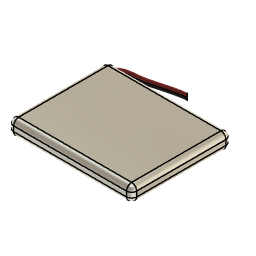
Bobblestat_rev2_v22 (Autodesk Fusion 360 archive; units mm, degrees)
design "LiPo Battery Dummy"
Autodesk Fusion 360 part; units mm, degrees
sketch "Sketch1" plane through (0, 0, 0) normal (0, 0, 1) x (1, 0, 0)
  line L0 (0, 0) -> (36.5, 0)
  line L1 (36.5, 0) -> (36.5, 29.5)
  line L2 (36.5, 29.5) -> (0, 29.5)
  line L3 (0, 29.5) -> (0, 0)
  dimension "d1" = 36.5
  dimension "d2" = 29.5
  constraint horizontal L0
  constraint vertical L1
  constraint horizontal L2
  constraint vertical L3
  constraint coincident L0.start L3.end
  measures "d1" distance of L0.start L0.end
  measures "d2" distance of L0.start L2.end
extrude "Extrude1" add sketch "Sketch1" along normal blind 4.5
fillet "Fillet1" radius 1.5 4 edges at (0, 29.5, 2.25) (36.5, 0, 2.25) (0, 0, 2.25) (36.5, 29.5, 2.25) 2 faces at (12.1667, 9.8333, 4.5) (12.1667, 9.8333, 0)
ref_plane "WorkPlane1" through (18.25, 14.75, 1.5) normal (0, 0, -1) x (-1, 0, 0)
sketch "Sketch3" plane through (0, 0, 1.5) normal (0, 0, -1) x (-1, 0, 0)
  line L0 (-1.5, 29.5) -> (-1.5, 28)
  arc A0 (0, 28) -> (-1.5, 29.5) centre (-1.5, 28) ccw
  line L1 (-1.5, 28) -> (0, 28)
  spline S0 degree 5 poles (-1.5, 29.5) (-1.6067, 29.6112) (-1.8233, 29.824) (-2.1576, 30.1145) (-2.6223, 30.4444) (-3.2359, 30.7619) (-3.8851, 30.9901) (-4.5751, 31.1419) (-5.314, 31.2413) (-6.1112, 31.3189) (-6.9742, 31.4059) (-7.9068, 31.5288) (-8.9056, 31.7034) (-9.9588, 31.9304) (-11.0489, 32.2003) (-12.1553, 32.4969) (-13.2569, 32.8008) (-14.3343, 33.0926) (-15.3727, 33.3571) (-16.3632, 33.5849) (-17.3011, 33.7709) (-18.0079, 33.8846) (-18.5134, 33.95) (-18.8396, 33.9848) (-19, 34) knots 0 0 0 0 0 0 0.05 0.1 0.15 0.2 0.25 0.3 0.35 0.4 0.45 0.5 0.55 0.6 0.65 0.7 0.75 0.8 0.85 0.9 0.95 1 1 1 1 1 1
  point P0 (-4, 31)
  point P1 (-7.7183, 31.5108)
  point P2 (-14, 33)
  constraint coincident L0.start A0.end
sketch "Sketch4" plane through (0, 29.5, 0) normal (0, 1, 0) x (-1, 0, 0)
  line L0 (-1.5, 1.5) -> (-1.5, 3)
  line L1 (-1.5, 3) -> (-35, 3)
  line L2 (-35, 3) -> (-35, 1.5)
  line L3 (-35, 1.5) -> (-1.5, 1.5)
  circle A0 centre (-1.5, 2.7) radius 0.5
  circle A1 centre (-1.5, 1.8) radius 0.5
  dimension "d15" = 1
  dimension "d16" = 1
  dimension "d17" = 0.9
  dimension "d18" = 0.3
  constraint coincident L0 A0.centre
  constraint coincident L0 A1.centre
  measures "d15" diameter of A0
  measures "d16" diameter of A1
  measures "d17" distance of A0.centre A1.centre
  measures "d18" distance of L0.end A0.centre
sweep "Sweep1" add profiles "Sketch4" path "Sketch3" along S0 section 1 contours L0 L3 A0 A1 | L0 L3 A0 A1 | L0 A0 A1 | L0 A0 A1 | L0 L1 A0 A1 | L0 L1 A0 A1

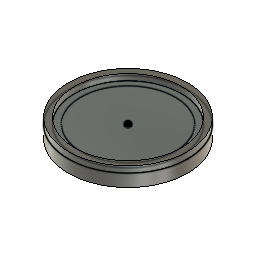
design "PCB sizing rev G"
Autodesk Fusion 360 part; units mm, degrees
sketch "Sketch1" plane through (0, 0, 0) normal (0, 0, 1) x (1, 0, 0)
  circle A0 centre (0, 0) radius 8.5
  circle A1 centre (0, 0) radius 7.5
  circle A2 centre (0, 0) radius 9.5
  dimension "d1" = 17
  dimension "d2" = 15
  dimension "d3" = 19
  constraint coincident A0.centre A1.centre
  constraint concentric A0 A1
  constraint concentric A1 A2
  measures "d1" diameter of A0
  measures "d2" diameter of A1
  measures "d3" diameter of A2
extrude "Extrude1" add sketch "Sketch1" against normal blind 2 contours A0 | A1 | A2
extrude "Extrude2" add sketch "Sketch1" along normal blind 1 contours A2
